tension_arm (Autodesk Fusion 360 design; units mm, degrees)
Autodesk Fusion 360 part; units mm, degrees
sketch "Sketch1" plane through (0, 0, 0) normal (0, 0, 1) x (1, 0, 0)
  line L0 (4, 0) -> (4, 18)
  line L1 (4, 18) -> (9, 18)
  line L2 (9, 18) -> (9, 39)
  line L3 (9, 39) -> (5, 39)
  line L4 (5, 39) -> (5, 22)
  line L5 (5, 22) -> (-5, 22)
  line L6 (-5, 22) -> (-5, 39)
  line L7 (-5, 39) -> (-9, 39)
  line L8 (-9, 39) -> (-9, 18)
  line L9 (-9, 18) -> (-4, 18)
  line L10 (-4, 18) -> (-4, 0)
  line L11 (-4, 0) -> (4, 0)
  point P0 (0, 22)
  dimension "d1" = 10
  dimension "d2" = 17
  dimension "d3" = 4
  dimension "d4" = 18
  dimension "d5" = 4
  dimension "d6" = 8
  constraint perpendicular L0 L1
  constraint perpendicular L1 L2
  constraint perpendicular L2 L3
  constraint perpendicular L3 L4
  constraint perpendicular L2 L5
  constraint perpendicular L3 L6
  constraint perpendicular L2 L7
  constraint perpendicular L7 L8
  constraint perpendicular L8 L9
  constraint midpoint L5 P0
  constraint horizontal L9
  constraint vertical origin P0
  constraint perpendicular L9 L10
  constraint horizontal L11
  constraint midpoint origin L11
  constraint equal L3 L7
  constraint collinear L3 L7
  constraint collinear L1 L9
  measures "d1" distance of L4 L6
  measures "d2" distance of L3 L5
  measures "d3" distance of L2 L4
  measures "d4" distance of L0.start L0.end
  measures "d5" distance of L1 L5
  measures "d6" distance of L0 L10
extrude "Extrude1" add sketch "Sketch1" along normal blind 15
sketch "Sketch2" plane through (-9, 0, 0) normal (-1, 0, 0) x (0, -1, 0)
  line L0 (-39, 0) -> (-18, 0)
  line L1 (-18, 0) -> (-18, 15)
  line L2 (-18, 15) -> (-39, 15)
  line L3 (-39, 15) -> (-39, 0)
  circle A0 centre (-32, 7.5) radius 1.6
  line L4 (-22, 0) -> (-22, 15)
  line L5 (-8.8, 11.1) -> (-5, 11.1)
  line L6 (-5, 11.1) -> (-5, 3.9)
  line L7 (-5, 3.9) -> (-8.8, 3.9)
  line L8 (-8.8, 3.9) -> (-8.8, 11.1)
  line L9 (-8.8, 11.1) -> (-5, 3.9) construction
  line L10 (-5, 11.1) -> (-8.8, 3.9) construction
  line L11 (0, 0) -> (0, 15)
  point P0 (-39, 7.5)
  point P1 (-6.9, 7.5)
  point P2 (0, 7.5)
  dimension "d9" = 3.2
  dimension "d11" = 10
  dimension "d18" = 7.2
  dimension "d19" = 3.8
  dimension "d20" = 5
  constraint midpoint L3 P0
  constraint horizontal A0.centre P0
  constraint perpendicular L5 L6
  constraint parallel L5 L7
  constraint parallel L6 L8
  constraint horizontal L5
  constraint coincident L9 P1
  constraint coincident L10 P1
  constraint midpoint L11 P2
  constraint horizontal P1 P2
  measures "d9" diameter of A0
  measures "d11" distance of A0.centre L4
  measures "d18" distance of L5.end L6.end
  measures "d19" distance of L5.start L5.end
  measures "d20" distance of L6 L11
extrude "Extrude2" cut sketch "Sketch2" against normal up to surface (18 mm away) contours A0 | L5 L6 L7 L8
ref_plane "WorkPlane1" through (0, 19.5, 7.5) normal (0, 0, 1) x (1, 0, 0)
sketch "Sketch4" plane through (0, 17, 7.5) normal (0, 0, 1) x (1, 0, 0)
  line L0 (-5, 16.6) -> (-5, 13.4)
  line L1 (-9, 13.4) -> (-9, 16.6)
  line L2 (9, 16.6) -> (9, 13.4)
  line L3 (5, 13.4) -> (5, 16.6)
  line L4 (-9, 15) -> (9, 15) construction
  line L5 (-5, 13.4) -> (-5, 11.9)
  line L6 (-5, 11.9) -> (-4.25, 12.9)
  line L7 (-4.25, 12.9) -> (-4.25, 13.4)
  line L8 (-4.25, 13.4) -> (-5, 13.4)
  line L9 (5, 13.4) -> (5, 11.9)
  line L10 (5, 11.9) -> (4.25, 12.9)
  line L11 (4.25, 12.9) -> (4.25, 13.4)
  line L12 (4.25, 13.4) -> (5, 13.4)
  dimension "d14" = 0.75
  dimension "d15" = 0.5
  dimension "d16" = 1.5
  constraint midpoint L1 L4.start
  constraint midpoint L2 L4.end
  constraint coincident L0.end L5.start
  constraint parallel L0 L5
  constraint parallel L5 L7
  constraint perpendicular L5 L8
  constraint coincident L3.start L9.start
  constraint perpendicular L8 L9
  constraint parallel L9 L11
  constraint perpendicular L9 L12
  constraint horizontal L6.end L10.end
  constraint horizontal L5.end L9.end
  constraint equal L8 L12
  measures "d14" distance of L0.end L7.end
  measures "d15" distance of L6.end L7.end
  measures "d16" distance of L0.end L5.end
revolve "Revolve1" add sketch "Sketch4" angle 360 about axis through (-9, 32, 7.5) along (1, 0, 0)
sketch "Sketch5" plane through (0, 0, 0) normal (0, -1, 0) x (1, 0, 0)
  line L0 (-4, 0) -> (4, 0)
  line L1 (4, 0) -> (4, 15)
  line L2 (4, 15) -> (-4, 15)
  line L3 (-4, 15) -> (-4, 0)
  circle A0 centre (0, 7.5) radius 2.1
  point P0 (-4, 7.5)
  dimension "d21" = 4.2
  constraint midpoint L3 P0
  constraint horizontal A0.centre P0
  constraint vertical origin A0.centre
  measures "d21" diameter of A0
extrude "Extrude3" cut sketch "Sketch5" against normal blind 19 contours A0
fillet "Fillet1" radius 3 4 edges at (-9, 18, 7.5) (-9, 39, 7.5) (9, 39, 7.5) (9, 18, 7.5)
chamfer "Chamfer1" distance 1 angle 45 4 edges at (0, 0, 15) (-4, 0, 7.5) (0, 0, 0) (4, 0, 7.5)
sketch "Sketch6" plane through (-9, 0, 0) normal (-1, 0, 0) x (0, -1, 0)
  circle A0 centre (-32, 7.5) radius 1.6
  line L0 (-36, 15) -> (-36, 0)
  line L1 (-36, 0) -> (-21, 0)
  line L2 (-21, 0) -> (-21, 15)
  line L3 (-21, 15) -> (-36, 15)
  line L4 (-33.6454, 10.35) -> (-35.2909, 7.5)
  line L5 (-35.2909, 7.5) -> (-33.6454, 4.65)
  line L6 (-33.6454, 4.65) -> (-30.3546, 4.65)
  line L7 (-30.3546, 4.65) -> (-28.7091, 7.5)
  line L8 (-28.7091, 7.5) -> (-30.3546, 10.35)
  line L9 (-30.3546, 10.35) -> (-33.6454, 10.35)
  point P0 (-32, 7.5)
  dimension "d50" = 5.7
  constraint coincident P0 A0.centre
  constraint horizontal L9
  measures "d50" distance of L6 L9
extrude "Extrude4" cut sketch "Sketch6" against normal blind 2 contours L4 L5 L6 L7 L8 L9
sketch "Sketch7" plane through (9, 0, 0) normal (1, 0, 0) x (0, 1, 0)
  circle A0 centre (32, 7.5) radius 1.6
  line L0 (21, 15) -> (21, 0)
  line L1 (21, 0) -> (36, 0)
  line L2 (36, 0) -> (36, 15)
  line L3 (36, 15) -> (21, 15)
  circle A1 centre (32, 7.5) radius 3
  dimension "d53" = 6
  constraint concentric A0 A1
  measures "d53" diameter of A1
extrude "Extrude5" cut sketch "Sketch7" against normal blind 2 contours A1
